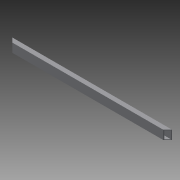
# Autodesk Inventor part: 36in 2x1 double corner
Saved by Autodesk Inventor 2015 (Build 190159000, 159)
## iProperties
Created: 2015-01-12
Part Number: 36in 2x1 double corner
Material: Generic
Document SubType Name: Modeling
Designer: whitaus15
Density: 1 g/cm^3
Appearance: Default
Author: whitaus15
Autodesk Inventor part; units mm, degrees
ref_plane "YZ Plane" through (0, 0, 0) normal (1, 0, 0) x (0, 1, 0)
ref_plane "XZ Plane" through (0, 0, 0) normal (0, 1, 0) x (-1, 0, 0)
sketch "Sketch1" plane through (0, 0, 0) normal (0, 1, 0) x (-1, 0, 0)
  line L0 (0, 0) -> (914.4, 0)
  line L1 (914.4, 0) -> (914.4, 25.4)
  line L2 (914.4, 25.4) -> (889, 25.4)
  line L3 (889, 25.4) -> (914.4, 0)
  line L4 (889, 25.4) -> (25.4, 25.4)
  line L5 (25.4, 25.4) -> (0, 0)
  dimension "d0" = 914.4
  dimension "d1" = 25.4
  dimension "d2" = 25.4
  dimension "d3" = 863.6
  constraints: 12 end point, 2 horizontal, 1 point on line, 1 vertical
  measures "d0" distance of L0.start L0.end
  measures "d1" distance of L0.end L1.end
  measures "d2" distance of L1.end L2.end
  measures "d3" distance of L2.end L4.end
extrude "Extrusion1" add sketch "Sketch1" along normal blind 50.8 contours L5 L4 L3 L0
ref_plane "Work Plane1" through (-457.2, 0, 457.2) normal (1, 0, 0) x (0, 1, 0)
sketch "Sketch2" plane through (-457.2, 0, 457.2) normal (1, 0, 0) x (0, 1, 0)
  line L0 (50.8, -457.2) -> (47.625, -457.2)
  line L1 (0, -457.2) -> (50.8, -457.2) projected
  line L2 (47.625, -457.2) -> (47.625, -454.025)
  line L3 (47.625, -454.025) -> (3.175, -454.025)
  line L4 (3.175, -454.025) -> (3.175, -434.975)
  line L5 (3.175, -434.975) -> (47.625, -434.975)
  line L6 (47.625, -434.975) -> (47.625, -454.025)
  dimension "d6" = 3.175
  dimension "d7" = 3.175
  dimension "d8" = 44.45
  dimension "d9" = 19.05
  constraints: 12 end point, 2 parallel, 2 perpendicular, 1 horizontal, 1 point on line
  measures "d6" distance of L0.start L0.end
  measures "d7" distance of L0.end L2.end
  measures "d8" distance of L4.end L5.end
  measures "d9" distance of L3.end L4.end
extrude "Extrusion2" cut sketch "Sketch2" along normal through all both and the other way through all
body "Solid1"
